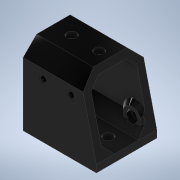
# Autodesk Inventor part: Soporte Actuador
Saved by Autodesk Inventor 2022 (Build 260153000, 153)
## iProperties
Created: 2021-02-18
Part Number: Soporte Actuador
Material: PET Plastic
Document SubType Name: Modeling
Designer: juanp
Density: 1.541 g/cm^3
Appearance: Polycarbonate - Clear
Author: juanp
Autodesk Inventor part; units mm, degrees
ref_plane "YZ Plane" through (0, 0, 0) normal (1, 0, 0) x (0, 1, 0)
ref_plane "XZ Plane" through (0, 0, 0) normal (0, 1, 0) x (-1, 0, 0)
ref_plane "XY Plane" through (0, 0, 0) normal (0, 0, 1) x (1, 0, 0)
sketch "Sketch18" plane through (0, 0, 0) normal (0, 1, 0) x (-1, 0, 0)
  circle A0 centre (10, 0) radius 2.65
  circle A1 centre (-10, 0) radius 2.65
  line L0 (10, 0) -> (-10, 0)
  line L1 (20, -16.5) -> (-20, -16.5)
  line L2 (-20, -16.5) -> (-20, 16.5)
  line L3 (-20, 16.5) -> (20, 16.5)
  line L4 (20, 16.5) -> (20, -16.5)
  line L5 (-20, 12.5) -> (16, 12.5)
  line L6 (16, 12.5) -> (16, -12.5)
  line L7 (16, -12.5) -> (-20, -12.5)
  circle A2 centre (10, 0) radius 4.75 construction
  circle A3 centre (-10, 0) radius 4.75 construction
  point P0 (0, 0)
  point P1 (0, 0)
  dimension "d92" = 5.3
  dimension "d93" = 20
  dimension "d94" = 16.5
  dimension "d95" = 16.5
  dimension "d96" = 10
  dimension "d97" = 10
  dimension "d100" = 4
  dimension "d101" = 4
  dimension "d102" = 4
  dimension "d111" = 9.5
  constraints: 16 end point, 4 centre point, 3 coincident, 3 horizontal, 3 perpendicular, 2 equal radius, 2 parallel, 2 point on line, 1 midpoint
  measures "d92" diameter of A0
  measures "d93" distance of L0.start L0.end
  measures "d94" distance between parallel lines of L1 L0
  measures "d95" distance between parallel lines of L3 L0
  measures "d96" distance from line of L4 L0.start
  measures "d97" distance from line of L2 L0.end
  measures "d100" distance between parallel lines of L1 L7
  measures "d101" distance between parallel lines of L4 L6
  measures "d102" distance between parallel lines of L3 L5
  measures "d111" diameter of A3
extrude "Extrusion21" add sketch "Sketch18" along normal blind 4
extrude "Extrusion22" add sketch "Sketch18" along normal blind 42 contours L1 L2 L7 L6 L5 L3 L4
sketch "Sketch19" plane through (0, 42, 0) normal (0, 1, 0) x (1, 0, 0)
  line L0 (-20, 16.5) -> (-20, -16.5) projected
  line L1 (-20, -16.5) -> (20, -16.5) projected
  line L2 (20, -16.5) -> (20, -12.5) projected
  line L3 (20, -12.5) -> (-16, -12.5) projected
  line L4 (-16, -12.5) -> (-16, 12.5) projected
  line L5 (-16, 12.5) -> (20, 12.5) projected
  line L6 (20, 12.5) -> (20, 16.5) projected
  line L7 (20, 16.5) -> (-20, 16.5) projected
  line L8 (-16, 12.5) -> (-16, -12.5) projected
  line L9 (20, -16.5) -> (20, 16.5) projected
  circle A0 centre (-10, 0) radius 2.65 projected
  circle A1 centre (5, 0) radius 2.65
  line L10 (5, 0) -> (-10, 0) construction
  line L11 (-20, -16.5) -> (20, -16.5) projected
  line L12 (11, -16.5) -> (11, 16.5)
  line L13 (-20, 16.5) -> (-20, -16.5) projected
  line L14 (5, 0) -> (11, 0) construction
  line L15 (-10, 0) -> (-16, 0) construction
  point P0 (0, 0)
  point P1 (11, -12.5)
  point P2 (11, 12.5)
  dimension "d126" = 15
  constraints: 8 end point, 2 horizontal, 2 midpoint, 2 point on line, 1 centre point, 1 collinear, 1 equal radius, 1 perpendicular
  measures "d126" distance of L10.start L10.end
extrude "Extrusion23" add sketch "Sketch19" against normal blind 4 contours L12 L3 L4 L5
chamfer "Chamfer9" distance 9 distance2 38 1 edges at (20, 42, 14.5) measured on face at (19.5, 42, 14.5)
chamfer "Chamfer10" distance 9 distance2 38 1 edges at (20, 42, -14.5) measured on face at (19.5, 42, -14.5)
chamfer "Chamfer6" distance 6 angle 45 2 edges at (2, 4, -12.5) (2, 4, 12.5)
chamfer "Chamfer7" distance 5 angle 45 2 edges at (-2.5, 38, 12.5) (-2.5, 38, -12.5)
chamfer "Chamfer8" distance 7.343 angle 45 2 edges at (-4.5, 42, 16.5) (-4.5, 42, -16.5)
sketch "Sketch22" plane through (0, 38, 0) normal (0, -1, 0) x (1, 0, 0)
  circle A0 centre (-10, 0) radius 2.65 projected
  line L0 (7.65, 7.5) -> (7.65, -7.5)
  line L1 (2.35, 7.5) -> (2.35, -7.5)
  line L2 (-7.35, 7.5) -> (-7.35, -7.5)
  line L3 (-12.65, -7.5) -> (-12.65, 7.5)
  line L4 (7.65, 2.65) -> (2.35, 2.65)
  line L5 (-7.35, 2.65) -> (-12.65, 2.65)
  line L6 (-12.65, -2.65) -> (-7.35, -2.65)
  line L7 (2.35, -2.65) -> (7.65, -2.65)
  line L8 (11.9474, 12.5) -> (11, 12.5) projected
  line L9 (11, -12.5) -> (11.9474, -12.5) projected
  circle A1 centre (5, 0) radius 2.65 projected
  line L10 (11.9474, 13.157) -> (11.9474, 12.5) projected
  line L11 (11.9474, -12.5) -> (11.9474, -13.157) projected
  line L12 (11, 12.5) -> (11, 7.5) projected
  line L13 (11, 7.5) -> (-16, 7.5) projected
  line L14 (-16, 7.5) -> (-16, -7.5) projected
  line L15 (-16, -7.5) -> (11, -7.5) projected
  line L16 (11, -7.5) -> (11, -12.5) projected
  line L17 (11.9474, -13.157) -> (-20, -13.157) projected
  line L18 (-20, -13.157) -> (-20, 13.157) projected
  line L19 (-20, 13.157) -> (11.9474, 13.157) projected
  line L20 (11, 7.5) -> (11, -7.5) projected
  point P0 (0, 0)
  point P1 (-10, -2.65)
  point P2 (-12.65, 0)
  point P3 (-10, 2.65)
  point P4 (-7.35, 0)
  point P5 (5, 2.65)
  point P6 (7.65, 0)
  point P7 (5, -2.65)
  point P8 (2.35, 0)
  constraints: 16 end point, 12 point on line, 8 tangent, 3 equal length, 2 perpendicular, 2 vertical, 1 horizontal
extrude "Extrusion24" cut sketch "Sketch22" against normal blind 0.3 contours L5 L3 L13 L2 | L6 L2 L15 L3 | L13 L0 L4 L1 | L1 L7 L0 L15
extrude "Extrusion25" cut sketch "Sketch22" against normal blind 0.6 contours L2 L6 A0 | A0 L5 L2 | A0 L3 L5 | L6 L3 A0 | L4 A1 L1 | L1 A1 L7 | L4 L0 A1 | A1 L0 L7
sketch "Sketch23" plane through (11, 38, 7.5) normal (1, 0, 0) x (0, 0, -1)
  line L0 (16.657, 4) -> (20, 0.657) projected
  line L1 (-1.657, 4) -> (16.657, 4) projected
  line L2 (-5, 0.657) -> (-1.657, 4) projected
  line L3 (-5, -5) -> (-5, 0.657) projected
  line L4 (0, 0) -> (-5, -5) projected
  line L5 (15, 0) -> (0, 0) projected
  line L6 (20, -5) -> (15, 0) projected
  line L7 (20, 0.657) -> (20, -5) projected
  point P0 (7.5, -38)
extrude "Extrusion26" add sketch "Sketch23" along normal up to surface surface through (15.5, 23, 8.25) normal (0.9730803, 0.2304664, 0)
sketch "Sketch24" plane through (20, 0, -16.5) normal (0, 0, -1) x (-1, 0, 0)
  line L0 (7.3, 0) -> (7.3, 9.76) construction
  line L1 (7.3, 9.76) -> (40, 9.76) construction
  line L2 (40, 0) -> (40, 34.657) projected
  line L3 (0, 0) -> (40, 0) construction
  circle A0 centre (7.3, 9.76) radius 1.65
  point P0 (20, 0)
  dimension "d135" = 9.76
  dimension "d136" = 32.7
  dimension "d137" = 3.3
  constraints: 4 end point, 2 point on line, 1 centre point, 1 coincident, 1 horizontal, 1 vertical
  measures "d135" distance of L0.start L0.end
  measures "d136" distance of L0.end L1.end
  measures "d137" diameter of A0
extrude "Extrusion27" cut sketch "Sketch24" against normal blind 10
sketch "Sketch25" plane through (-16, 33, -12.5) normal (0, 0, 1) x (1, 0, 0)
  circle A0 centre (28.7, -23.24) radius 1.65 projected
  line L0 (25.4553, -23.24) -> (27.0776, -20.43)
  line L1 (27.0776, -20.43) -> (30.3224, -20.43)
  line L2 (30.3224, -20.43) -> (31.9447, -23.24)
  line L3 (31.9447, -23.24) -> (30.3224, -26.05)
  line L4 (30.3224, -26.05) -> (27.0776, -26.05)
  line L5 (27.0776, -26.05) -> (25.4553, -23.24)
  circle A1 centre (28.7, -23.24) radius 4.7447
  line L6 (25.4553, -23.24) -> (23.9553, -23.24) construction
  point P0 (16, -33)
  dimension "d141" = 5.62
  dimension "d146" = 1.5
  constraints: 14 end point, 2 coincident, 2 horizontal, 1 horizontal alignment, 15 other
  measures "d141" distance between parallel lines of L0 L3
  measures "d146" distance of L0.start L6.end
extrude "Extrusion28" cut sketch "Sketch25" along normal blind 10 contours A0 | L0 L1 L2 L3 L4 L5
extrude "Extrusion29" add sketch "Sketch25" along normal blind 2.35 contours A1
sketch "Sketch26" plane through (-20, 0, 16.5) normal (0, 0, 1) x (1, 0, 0)
  line L0 (4, 33) -> (33.1316, 33) construction
  line L1 (38.5789, 10) -> (33.1316, 33) construction
  line L2 (4, 10) -> (38.5789, 10) construction
  line L3 (4, 10) -> (4, 33) construction
  line L4 (4, 10) -> (4, 33) construction
  line L5 (4, 10) -> (33.1316, 33) construction
  line L6 (8.0658, 34.3285) -> (29.0658, 34.3285) construction
  line L7 (29.0658, 34.3285) -> (29.0658, 0.3285) construction
  line L8 (29.0658, 0.3285) -> (8.0658, 0.3285) construction
  line L9 (8.0658, 0.3285) -> (8.0658, 34.3285) construction
  line L10 (8.0658, 34.3285) -> (29.0658, 0.3285) construction
  line L11 (29.0658, 34.3285) -> (8.0658, 0.3285) construction
  line L12 (33.1316, 33) -> (4, 33) construction
  line L13 (27.9614, 10) -> (4, 10) construction
  line L14 (0, 0) -> (0, 34.657) construction
  line L15 (33.1316, 33) -> (38.5789, 10) construction
  line L16 (38.5789, 10) -> (33.1316, 33) construction
  line L17 (18.5658, 21.5) -> (18.5658, 17.3285) construction
  line L18 (18.1534, 0.3285) -> (18.1534, 0) construction
  line L19 (18.5658, 34.3285) -> (18.5658, 34.657) construction
  line L20 (0, 0) -> (40, 0) construction
  line L21 (0, 34.657) -> (32.7391, 34.657) construction
  line L22 (18.5658, 34.3285) -> (18.5658, 29.9535) construction
  line L23 (10.9659, 29.9535) -> (26.1657, 29.9535) construction
  circle A0 centre (10.9659, 29.9535) radius 1.65
  circle A1 centre (26.1657, 29.9535) radius 1.65
  point P0 (18.5658, 17.3285)
  dimension "d153" = 34
  dimension "d154" = 21
  dimension "d155" = 4.375
  dimension "d156" = 3.3
  dimension "d157" = 15.1998
  constraints: 24 end point, 6 midpoint, 3 parallel, 3 point on line, 3 vertical, 2 centre point, 2 coincident, 2 horizontal, 2 perpendicular, 1 equal radius
  measures "d153" distance of L6.end L7.end
  measures "d154" distance of L7.end L8.end
  measures "d155" distance of L22.end L19.start
  measures "d156" diameter of A1
  measures "d157" distance of L23.start L23.end
extrude "Extrusion30" cut sketch "Sketch26" against normal blind 10
sketch "Sketch27" plane through (18.5789, 10, 12.5) normal (0, 0, -1) x (-1, 0, 0)
  line L0 (24.3683, 19.9535) -> (25.9907, 22.7635)
  line L1 (25.9907, 22.7635) -> (29.2354, 22.7635)
  line L2 (29.2354, 22.7635) -> (30.8578, 19.9535)
  line L3 (30.8578, 19.9535) -> (29.2354, 17.1435)
  line L4 (29.2354, 17.1435) -> (25.9907, 17.1435)
  line L5 (25.9907, 17.1435) -> (24.3683, 19.9535)
  circle A0 centre (27.6131, 19.9535) radius 4.7447
  line L6 (24.3683, 19.9535) -> (22.8683, 19.9535) construction
  circle A1 centre (12.4133, 19.9535) radius 1.65 projected
  circle A2 centre (27.6131, 19.9535) radius 1.65 projected
  line L7 (9.1685, 19.9535) -> (10.7909, 22.7635)
  line L8 (10.7909, 22.7635) -> (14.0356, 22.7635)
  line L9 (14.0356, 22.7635) -> (15.658, 19.9535)
  line L10 (15.658, 19.9535) -> (14.0356, 17.1435)
  line L11 (14.0356, 17.1435) -> (10.7909, 17.1435)
  line L12 (10.7909, 17.1435) -> (9.1685, 19.9535)
  circle A3 centre (12.4133, 19.9535) radius 4.7447
  line L13 (9.1685, 19.9535) -> (7.6685, 19.9535) construction
  point P0 (18.5789, -10)
  dimension "d160" = 5.62
  dimension "d161" = 1.5
  dimension "d162" = 5.62
  dimension "d163" = 1.5
  constraints: 28 end point, 4 coincident, 4 horizontal, 2 horizontal alignment, 30 other
  measures "d160" distance between parallel lines of L0 L3
  measures "d161" distance of L0.start L6.end
  measures "d162" distance between parallel lines of L7 L10
  measures "d163" distance of L7.start L13.end
extrude "Extrusion31" add sketch "Sketch27" along normal blind 2.35 contours A0 | A3
chamfer "Chamfer12" distance 2.35 angle 45 5 edges at (1.7064, 31.5742, 12.5) (7.7864, 25.4942, 12.5) (-13.4934, 31.5742, 12.5) (-7.4134, 25.4942, 12.5) (12.7, 14.5047, -12.5)
body "Solid3"
